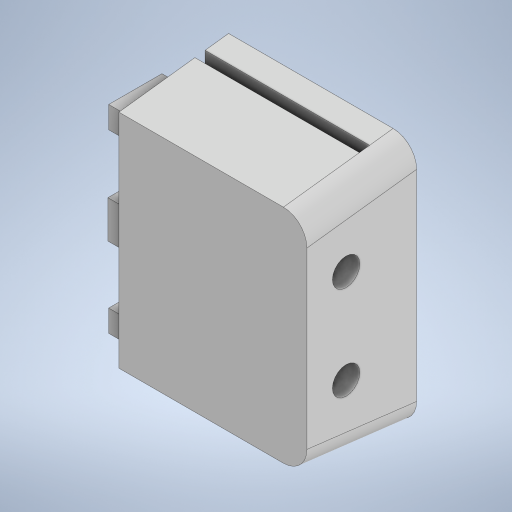
# Autodesk Inventor part: finlay_holds_down
Saved by Autodesk Inventor 2024 (Build 280153000, 153)
## iProperties
Created: 2024-09-23
Part Number: finlay_holds_down
Material: 一般
Document SubType Name: Modeling
Designer: 1412z
Density: 1 g/cm^3
Appearance: 既定
Author: 1412z
Autodesk Inventor part; units mm, degrees
ref_plane "YZ Plane" through (0, 0, 0) normal (1, 0, 0) x (0, 1, 0)
ref_plane "XZ Plane" through (0, 0, 0) normal (0, 1, 0) x (-1, 0, 0)
ref_plane "XY Plane" through (0, 0, 0) normal (0, 0, 1) x (1, 0, 0)
sketch "スケッチ1" plane through (0, 0, 0) normal (1, 0, 0) x (0, 1, 0)
  line L0 (0, 0) -> (31.7, 0)
  line L1 (1.7, 14) -> (30, 14)
  line L2 (1.7, 14) -> (0, 0)
  line L3 (30, 14) -> (31.7, 0)
  dimension "d0" = 31.7
  dimension "d1" = 28.3
  constraints: 8 end point, 2 horizontal
  measures "d0" distance of L0.start L0.end
  measures "d1" distance of L1.start L1.end
extrude "押し出し1" add sketch "スケッチ1" against normal blind 24
sketch "スケッチ2" plane through (-24, 0, 0) normal (-1, 0, 0) x (0, 0, 1)
  line L0 (0, 0) -> (14, 1.7) projected
  line L1 (3, 0.3643) -> (3, 31.3357)
  line L2 (14, 30) -> (0, 31.7) projected
  line L3 (4.3, 0.3643) -> (4.3, 31.3357)
  line L4 (4.3, 31.3357) -> (3, 31.3357)
  line L5 (4.3, 0.3643) -> (3, 0.3643)
  point P0 (4.3, 0.5221)
  point P1 (4.3, 31.1779)
  constraints: 8 end point, 2 point on line, 2 vertical, 1 parallel, 1 perpendicular
extrude "押し出し2" cut sketch "スケッチ2" against normal blind 21 contours L1 L2 L3 L0
sketch "スケッチ4" plane through (-3, 0, 0) normal (-1, 0, 0) x (0, 0, 1)
  circle A0 centre (9, 9.85) radius 1.75
  circle A1 centre (9, 21.85) radius 1.75
  point P0 (0, 0)
  dimension "d10" = 3.5
  dimension "d11" = 3.5
  constraints: 2 centre point
  measures "d10" diameter of A0
  measures "d11" diameter of A1
extrude "押し出し4" cut sketch "スケッチ4" along normal mid plane 100
fillet "フィレット1" radius 3 2 edges at (0, 30.85, 7) (0, 0.85, 7)
sketch "スケッチ10" plane through (-24, 0, 0) normal (-1, 0, 0) x (0, 0, 1)
  line L0 (5.6, 13.45) -> (12.4, 13.45)
  line L1 (12.4, 13.45) -> (12.4, 18.25)
  line L2 (12.4, 18.25) -> (5.6, 18.25)
  line L3 (5.6, 18.25) -> (5.6, 13.45)
  line L4 (5.6, 13.45) -> (12.4, 18.25) construction
  line L5 (12.4, 13.45) -> (5.6, 18.25) construction
  line L6 (14, 1.7) -> (14, 30) projected
  point P0 (0, 0)
  point P1 (9, 15.85)
  point P2 (14, 15.85)
  dimension "d29" = 6.8
  dimension "d30" = 4.8
  dimension "d44" = 5
  constraints: 12 end point, 3 midpoint, 2 parallel, 1 horizontal, 1 perpendicular
  measures "d29" distance of L2.end L1.end
  measures "d30" distance of L1.end L0.end
  measures "d44" distance of point (9, 15.85) point (14, 15.85)
extrude "押し出し10" add sketch "スケッチ10" along normal blind 3
sketch "スケッチ11" plane through (-24, 0, 0) normal (-1, 0, 0) x (0, 0, 1)
  line L0 (12.3, 3.2) -> (5.5, 3.2)
  line L1 (5.5, 3.2) -> (5.5, 6)
  line L2 (5.5, 6) -> (12.3, 6)
  line L3 (12.3, 6) -> (12.3, 3.2)
  line L4 (12.3, 3.2) -> (5.5, 6) construction
  line L5 (5.5, 3.2) -> (12.3, 6) construction
  line L6 (12.3, 28.5) -> (5.5, 28.5)
  line L7 (5.5, 28.5) -> (5.5, 25.7)
  line L8 (5.5, 25.7) -> (12.3, 25.7)
  line L9 (12.3, 25.7) -> (12.3, 28.5)
  line L10 (12.3, 28.5) -> (5.5, 25.7) construction
  line L11 (5.5, 28.5) -> (12.3, 25.7) construction
  point P0 (0, 0)
  point P1 (8.9, 4.6)
  point P2 (8.9, 27.1)
  dimension "d33" = 6.8
  dimension "d34" = 2.8
  dimension "d35" = 6.8
  dimension "d36" = 2.8
  constraints: 24 end point, 4 midpoint, 4 parallel, 2 horizontal, 2 perpendicular
  measures "d33" distance of L1.end L2.end
  measures "d34" distance of L0.end L1.end
  measures "d35" distance of L8.end L7.end
  measures "d36" distance of L7.end L6.end
extrude "押し出し11" add sketch "スケッチ11" along normal blind 3
sketch "スケッチ12" plane through (-24, 0, 0) normal (-1, 0, 0) x (0, 0, 1)
  line L0 (2.05, 24.15) -> (0.75, 24.15)
  line L1 (0.75, 24.15) -> (0.75, 19.35)
  line L2 (0.75, 19.35) -> (2.05, 19.35)
  line L3 (2.05, 19.35) -> (2.05, 24.15)
  line L4 (2.05, 24.15) -> (0.75, 19.35) construction
  line L5 (0.75, 24.15) -> (2.05, 19.35) construction
  line L6 (0.75, 7.45) -> (2.05, 7.45)
  line L7 (2.05, 7.45) -> (2.05, 12.25)
  line L8 (2.05, 12.25) -> (0.75, 12.25)
  line L9 (0.75, 12.25) -> (0.75, 7.45)
  line L10 (0.75, 7.45) -> (2.05, 12.25) construction
  line L11 (2.05, 7.45) -> (0.75, 12.25) construction
  point P0 (0, 0)
  point P1 (1.4, 21.75)
  point P2 (1.4, 9.85)
  dimension "d39" = 1.3
  dimension "d40" = 4.8
  dimension "d45" = 1.3
  dimension "d46" = 4.8
  constraints: 24 end point, 4 midpoint, 4 parallel, 2 horizontal, 2 perpendicular
  measures "d39" distance of L2.end L1.end
  measures "d40" distance of L1.end L0.end
  measures "d45" distance of L8.end L7.end
  measures "d46" distance of L7.end L6.end
extrude "押し出し12" add sketch "スケッチ12" along normal blind 3 contours L3 L2 L1 L0
sketch "スケッチ13" plane through (-24, 0, 0) normal (-1, 0, 0) x (0, 0, 1)
  line L0 (2.05, 12.25) -> (0.75, 12.25)
  line L1 (0.75, 12.25) -> (0.75, 7.45)
  line L2 (0.75, 7.45) -> (2.05, 7.45)
  line L3 (2.05, 7.45) -> (2.05, 12.25)
  line L4 (2.05, 12.25) -> (0.75, 7.45) construction
  line L5 (0.75, 12.25) -> (2.05, 7.45) construction
  point P0 (0, 0)
  point P1 (1.4, 9.85)
  dimension "d47" = 1.3
  dimension "d48" = 4.8
  constraints: 12 end point, 2 midpoint, 2 parallel, 1 horizontal, 1 perpendicular
  measures "d47" distance of L2.end L1.end
  measures "d48" distance of L1.end L0.end
extrude "押し出し13" add sketch "スケッチ13" along normal blind 3
